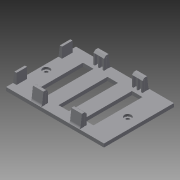
# Autodesk Inventor part: breadboard clip
Saved by Autodesk Inventor 2014 SP1 (Build 180222100, 222)
## iProperties
Created: 2017-08-14
Part Number: breadboard clip
Material: Generic
Document SubType Name: Modeling
Designer: kteo17
Density: 1 g/cm^3
Appearance: Default
Author: kteo17
Autodesk Inventor part; units mm, degrees
ref_plane "YZ Plane" through (0, 0, 0) normal (1, 0, 0) x (0, 1, 0)
ref_plane "XZ Plane" through (0, 0, 0) normal (0, 1, 0) x (-1, 0, 0)
ref_plane "XY Plane" through (0, 0, 0) normal (0, 0, 1) x (1, 0, 0)
sketch "Sketch1" plane through (0, 0, 0) normal (0, 1, 0) x (-1, 0, 0)
  line L0 (0, 0) -> (88.9, 0)
  line L1 (88.9, 0) -> (88.9, 63.5)
  line L2 (88.9, 63.5) -> (0, 63.5)
  line L3 (0, 63.5) -> (0, 0)
  line L4 (73.025, 53.975) -> (63.5, 53.975)
  line L5 (63.5, 53.975) -> (63.5, 9.525)
  line L6 (63.5, 9.525) -> (73.025, 9.525)
  line L7 (73.025, 9.525) -> (73.025, 53.975)
  line L8 (50.8, 53.975) -> (41.275, 53.975)
  line L9 (41.275, 53.975) -> (41.275, 9.525)
  line L10 (41.275, 9.525) -> (50.8, 9.525)
  line L11 (50.8, 9.525) -> (50.8, 53.975)
  line L12 (28.575, 53.975) -> (19.05, 53.975)
  line L13 (19.05, 53.975) -> (19.05, 9.525)
  line L14 (19.05, 9.525) -> (28.575, 9.525)
  line L15 (28.575, 9.525) -> (28.575, 53.975)
  dimension "d0" = 88.9
  dimension "d1" = 63.5
  constraints: 32 end point, 8 parallel, 4 horizontal, 4 perpendicular
  measures "d0" distance of L2.end L1.end
  measures "d1" distance of L1.end L0.end
extrude "Extrusion1" add sketch "Sketch1" along normal blind 3.175
sketch "Sketch2" plane through (0, 3.175, 0) normal (0, 1, 0) x (1, 0, 0)
  line L0 (-88.9, 0) -> (-88.9, -63.5) projected
  line L1 (-88.9, -6.35) -> (-85.725, -6.35)
  line L2 (-85.725, -6.35) -> (-85.725, -15.875)
  line L3 (-85.725, -15.875) -> (-88.9, -15.875)
  line L4 (-88.9, -15.875) -> (-88.9, -6.35)
  line L5 (-88.9, -47.625) -> (-85.725, -47.625)
  line L6 (-85.725, -47.625) -> (-85.725, -57.15)
  line L7 (-85.725, -57.15) -> (-88.9, -57.15)
  line L8 (-88.9, -57.15) -> (-88.9, -47.625)
  constraints: 16 end point, 4 parallel, 2 horizontal, 2 perpendicular, 2 point on line
extrude "Extrusion2" add sketch "Sketch2" along normal blind 9.525
sketch "Sketch3" plane through (-88.9, 3.175, 57.15) normal (0, 0, 1) x (1, 0, 0)
  line L0 (0, 9.525) -> (3.175, 9.525) projected
  line L1 (0, 0) -> (0, 9.525) projected
  line L2 (1.1938, 9.525) -> (0, 0)
  line L3 (0, 0) -> (0, 9.525)
  line L4 (0, 9.525) -> (1.1938, 9.525)
  point P0 (88.9, -3.175)
  constraints: 6 end point, 2 collinear, 1 point on line
extrude "Extrusion3" cut sketch "Sketch3" against normal blind 50.8
sketch "Sketch4" plane through (0, 3.175, 0) normal (0, 1, 0) x (1, 0, 0)
  line L0 (-88.9, -63.5) -> (0, -63.5) projected
  line L1 (0, 0) -> (-88.9, 0) projected
  line L2 (-66.675, 0) -> (-57.15, 0)
  line L3 (-57.15, 0) -> (-57.15, -3.9624)
  line L4 (-57.15, -3.9624) -> (-66.675, -3.9624)
  line L5 (-66.675, -3.9624) -> (-66.675, 0)
  line L6 (-31.75, 0) -> (-22.225, 0)
  line L7 (-22.225, 0) -> (-22.225, -3.9624)
  line L8 (-22.225, -3.9624) -> (-31.75, -3.9624)
  line L9 (-31.75, -3.9624) -> (-31.75, 0)
  line L10 (-66.675, -63.5) -> (-57.15, -63.5)
  line L11 (-57.15, -63.5) -> (-57.15, -59.5376)
  line L12 (-57.15, -59.5376) -> (-66.675, -59.5376)
  line L13 (-66.675, -59.5376) -> (-66.675, -63.5)
  line L14 (-31.75, -63.5) -> (-22.225, -63.5)
  line L15 (-22.225, -63.5) -> (-22.225, -59.5376)
  line L16 (-22.225, -59.5376) -> (-31.75, -59.5376)
  line L17 (-31.75, -59.5376) -> (-31.75, -63.5)
  constraints: 32 end point, 8 parallel, 4 horizontal, 4 perpendicular, 4 point on line
extrude "Extrusion4" add sketch "Sketch4" along normal blind 11.1252
sketch "Sketch5" plane through (-22.225, 3.175, 63.5) normal (1, 0, 0) x (0, 0, -1)
  line L0 (3.9624, 0) -> (0, 0) projected
  line L1 (3.9624, 0) -> (3.9624, 11.1252) projected
  line L2 (0, 11.1252) -> (3.9624, 11.1252) projected
  line L3 (0, 0) -> (0, 11.1252) projected
  line L4 (3.9624, 12.7) -> (2.1844, 12.7)
  line L5 (3.9624, -0.6232) -> (0.7874, -0.6232)
  line L6 (2.1844, 11.1252) -> (0.7874, 0)
  line L7 (0.7874, 0) -> (0, 0)
  line L8 (0, 0) -> (0, 11.1252)
  line L9 (0, 11.1252) -> (2.1844, 11.1252)
  line L10 (59.5376, 0) -> (63.5, 0)
  line L11 (59.5376, 0) -> (59.5376, 11.1252)
  line L12 (63.5, 11.1252) -> (59.5376, 11.1252)
  line L13 (63.5, 0) -> (63.5, 11.1252)
  line L14 (59.5376, 12.7) -> (61.3156, 12.7)
  line L15 (59.5376, -0.6232) -> (62.7126, -0.6232)
  line L16 (61.3156, 11.1252) -> (62.7126, 0)
  line L17 (62.7126, 0) -> (63.5, 0)
  line L18 (63.5, 0) -> (63.5, 11.1252)
  line L19 (63.5, 11.1252) -> (61.3156, 11.1252)
  point P0 (63.5, -3.175)
  dimension "d17" = 1.778
  dimension "d18" = 3.175
  constraints: 32 end point, 6 point on line, 3 collinear, 1 parallel, 1 perpendicular
  measures "d17" distance of L4.start L4.end
  measures "d18" distance of L5.start L5.end
extrude "Extrusion5" cut sketch "Sketch5" against normal blind 44.45 contours L0 L3 L2 L6 | L16 L12 L13 L10
fillet "Fillet1" radius 3.175 4 edges at (-61.9125, 3.175, 62.7126) (-26.9875, 3.175, 62.7126) (-26.9875, 3.175, 0.7874) (-61.9125, 3.175, 0.7874)
sketch "Sketch6" plane through (0, 14.3002, 0) normal (0, 1, 0) x (1, 0, 0)
  line L0 (-22.225, -59.5376) -> (-31.75, -59.5376) projected
  line L1 (-31.75, -59.5376) -> (-22.225, -59.5376)
  line L2 (-22.225, -59.5376) -> (-22.225, -57.15)
  line L3 (-22.225, -57.15) -> (-31.75, -57.15)
  line L4 (-31.75, -57.15) -> (-31.75, -59.5376)
  line L5 (-57.15, -59.5376) -> (-66.675, -59.5376)
  line L6 (-66.675, -59.5376) -> (-66.675, -57.15)
  line L7 (-66.675, -57.15) -> (-57.15, -57.15)
  line L8 (-57.15, -57.15) -> (-57.15, -59.5376)
  line L9 (-31.75, -2.1844) -> (-22.225, -2.1844)
  line L10 (-22.225, -2.1844) -> (-22.225, -3.9624)
  line L11 (-22.225, -3.9624) -> (-31.75, -3.9624)
  line L12 (-31.75, -3.9624) -> (-31.75, -2.1844)
  line L13 (-31.75, -3.9624) -> (-22.225, -3.9624)
  line L14 (-22.225, -3.9624) -> (-22.225, -6.35)
  line L15 (-22.225, -6.35) -> (-31.75, -6.35)
  line L16 (-31.75, -6.35) -> (-31.75, -3.9624)
  line L17 (-57.15, -3.9624) -> (-66.675, -3.9624)
  line L18 (-66.675, -3.9624) -> (-66.675, -6.35)
  line L19 (-66.675, -6.35) -> (-57.15, -6.35)
  line L20 (-57.15, -6.35) -> (-57.15, -3.9624)
  point P0 (0, 0)
  constraints: 40 end point, 4 parallel, 2 horizontal, 2 perpendicular, 2 point on line
extrude "Extrusion6" add sketch "Sketch6" against normal blind 1.6002 contours L0 L4 L3 L2 | L5 L6 L7 L8 | L11 L14 L15 L16 | L20 L19 L18 L17
sketch "Sketch7" plane through (-22.225, 3.175, 63.5) normal (1, 0, 0) x (0, 0, -1)
  line L0 (6.35, 11.1252) -> (6.35, 9.525) projected
  line L1 (2.1844, 11.1252) -> (6.35, 11.1252) projected
  line L2 (4.5974, 11.1252) -> (6.35, 9.525)
  line L3 (4.5974, 11.1252) -> (6.35, 11.1252)
  line L4 (6.35, 9.525) -> (6.35, 11.1252)
  line L5 (61.3156, 11.1252) -> (62.4649, 1.9722)
  arc A0 (62.4649, 1.9722) -> (63.5, 0) centre (65.6152, 2.3678) ccw
  line L6 (59.5376, 0) -> (63.5, 0)
  line L7 (59.5376, 0) -> (59.5376, 9.525)
  line L8 (57.15, 9.525) -> (59.5376, 9.525)
  line L9 (57.15, 11.1252) -> (57.15, 9.525)
  line L10 (61.3156, 11.1252) -> (57.15, 11.1252)
  line L11 (58.9026, 11.1252) -> (57.15, 9.525)
  line L12 (58.9026, 11.1252) -> (57.15, 11.1252)
  line L13 (57.15, 9.525) -> (57.15, 11.1252)
  point P0 (63.5, -3.175)
  constraints: 24 end point, 2 point on circle, 2 point on line, 1 centre point, 1 collinear, 1 perpendicular
extrude "Extrusion7" cut sketch "Sketch7" against normal blind 44.45 contours L0 L2 L1 | L11 L9 L10
sketch "Sketch8" plane through (0, 3.175, 0) normal (0, 1, 0) x (1, 0, 0)
  circle A0 centre (-84.1375, -31.75) radius 3.175
  circle A1 centre (-10.1219, -31.75) radius 3.1695
  dimension "d29" = 74.0156
  constraints: 2 centre point
  measures "d29" distance of A1.centre A0.centre
extrude "Extrusion8" cut sketch "Sketch8" against normal blind 1.905
sketch "Sketch9" plane through (0, 3.175, 0) normal (0, 1, 0) x (1, 0, 0)
  circle A0 centre (-10.1219, -31.75) radius 3.1695 projected
  circle A1 centre (-84.1375, -31.75) radius 3.175 projected
  circle A2 centre (-84.1375, -31.75) radius 1.5875
  circle A3 centre (-10.1219, -31.75) radius 1.5875
  constraints: 2 centre point, 2 coincident
extrude "Extrusion9" cut sketch "Sketch9" against normal blind 3.175 contours A2 | A3
sketch "Sketch10" plane through (0, 3.175, 0) normal (0, 1, 0) x (1, 0, 0)
  line L0 (-57.15, -3.9624) -> (-66.675, -3.9624) projected
  line L1 (-66.675, -6.35) -> (-66.675, -4.318)
  line L2 (-66.675, -6.35) -> (-65.4088, -6.35)
  line L3 (-65.4088, -6.35) -> (-65.4088, -4.318)
  line L4 (-65.4088, -4.318) -> (-66.675, -4.318)
  line L5 (-57.15, -6.35) -> (-57.15, -4.318)
  line L6 (-57.15, -4.318) -> (-58.4191, -4.318)
  line L7 (-58.4191, -4.318) -> (-58.4191, -6.35)
  line L8 (-58.4191, -6.35) -> (-57.15, -6.35)
  line L9 (-61.9125, -6.35) -> (-61.2819, -6.35)
  line L10 (-61.2819, -6.35) -> (-61.2819, -4.318)
  line L11 (-61.2819, -4.318) -> (-62.5539, -4.318)
  line L12 (-62.5539, -4.318) -> (-62.5539, -6.35)
  line L13 (-62.5539, -6.35) -> (-61.9125, -6.35)
  line L14 (-31.75, -3.9624) -> (-22.225, -3.9624)
  line L15 (-22.225, -6.35) -> (-22.225, -4.318)
  line L16 (-22.225, -6.35) -> (-23.4912, -6.35)
  line L17 (-23.4912, -6.35) -> (-23.4912, -4.318)
  line L18 (-23.4912, -4.318) -> (-22.225, -4.318)
  line L19 (-31.75, -6.35) -> (-31.75, -4.318)
  line L20 (-31.75, -4.318) -> (-30.4809, -4.318)
  line L21 (-30.4809, -4.318) -> (-30.4809, -6.35)
  line L22 (-30.4809, -6.35) -> (-31.75, -6.35)
  line L23 (-26.9875, -6.35) -> (-27.6181, -6.35)
  line L24 (-27.6181, -6.35) -> (-27.6181, -4.318)
  line L25 (-27.6181, -4.318) -> (-26.3461, -4.318)
  line L26 (-26.3461, -4.318) -> (-26.3461, -6.35)
  line L27 (-26.3461, -6.35) -> (-26.9875, -6.35)
  line L28 (-22.225, -59.5376) -> (-31.75, -59.5376)
  line L29 (-57.15, -59.5376) -> (-66.675, -59.5376)
  line L30 (-66.675, -57.15) -> (-66.675, -59.182)
  line L31 (-66.675, -57.15) -> (-65.4088, -57.15)
  line L32 (-65.4088, -57.15) -> (-65.4088, -59.182)
  line L33 (-65.4088, -59.182) -> (-66.675, -59.182)
  line L34 (-57.15, -57.15) -> (-57.15, -59.182)
  line L35 (-57.15, -59.182) -> (-58.4191, -59.182)
  line L36 (-58.4191, -59.182) -> (-58.4191, -57.15)
  line L37 (-58.4191, -57.15) -> (-57.15, -57.15)
  line L38 (-61.9125, -57.15) -> (-61.2819, -57.15)
  line L39 (-61.2819, -57.15) -> (-61.2819, -59.182)
  line L40 (-61.2819, -59.182) -> (-62.5539, -59.182)
  line L41 (-62.5539, -59.182) -> (-62.5539, -57.15)
  line L42 (-62.5539, -57.15) -> (-61.9125, -57.15)
  line L43 (-23.4912, -59.182) -> (-22.225, -59.182)
  line L44 (-23.4912, -57.15) -> (-23.4912, -59.182)
  line L45 (-22.225, -57.15) -> (-23.4912, -57.15)
  line L46 (-22.225, -57.15) -> (-22.225, -59.182)
  line L47 (-26.3461, -57.15) -> (-26.9875, -57.15)
  line L48 (-26.3461, -59.182) -> (-26.3461, -57.15)
  line L49 (-27.6181, -59.182) -> (-26.3461, -59.182)
  line L50 (-27.6181, -57.15) -> (-27.6181, -59.182)
  line L51 (-26.9875, -57.15) -> (-27.6181, -57.15)
  line L52 (-30.4809, -57.15) -> (-31.75, -57.15)
  line L53 (-30.4809, -59.182) -> (-30.4809, -57.15)
  line L54 (-31.75, -59.182) -> (-30.4809, -59.182)
  line L55 (-31.75, -57.15) -> (-31.75, -59.182)
  line L56 (-31.75, -59.5376) -> (-22.225, -59.5376)
  line L57 (-63.5, -53.975) -> (-73.025, -53.975) projected
  line L58 (-69.85, -57.15) -> (-69.85, -59.182)
  dimension "d34" = 2.032
  dimension "d40" = 2.032
  constraints: 114 end point, 7 perpendicular, 4 parallel, 1 collinear
  measures "d34" distance of L1.start L1.end
  measures "d40" distance of L58.start L58.end
extrude "Extrusion10" add sketch "Sketch10" along normal blind 9.4488
sketch "Sketch11" plane through (-22.225, 3.175, 59.182) normal (1, 0, 0) x (0, 0, -1)
  line L0 (2.032, 0) -> (0, 0) projected
  line L1 (2.032, 0) -> (2.032, 9.4488) projected
  line L2 (0, 0) -> (2.032, 0)
  line L3 (2.032, 0) -> (2.032, 0.1331)
  line L4 (2.032, 0.1331) -> (0, 0.1331)
  line L5 (0, 0.1331) -> (0, 0)
  line L6 (54.864, 0) -> (57.15, 0)
  line L7 (57.15, 0) -> (57.15, 9.4488)
  line L8 (57.15, 0) -> (54.864, 0)
  line L9 (54.864, 0) -> (54.864, 0.1331)
  line L10 (54.864, 0.1331) -> (57.15, 0.1331)
  line L11 (57.15, 0.1331) -> (57.15, 0)
  point P0 (59.182, -3.175)
  constraints: 20 end point, 2 parallel, 1 horizontal, 1 perpendicular, 1 point on line
extrude "Extrusion11" cut sketch "Sketch11" against normal blind 44.45
body "Solid1"
